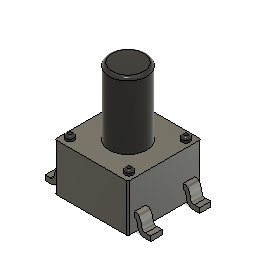
PTS 647 SK70 SMTR2 LFS v1 (Autodesk Fusion 360 design; units mm, degrees)
Autodesk Fusion 360 part; units mm, degrees
note: some values were not read from the file. Set by a fixed rule: which sketch regions a step uses.
sketch "Sketch1" plane through (0, 0, 0) normal (0, 1, 0) x (1, 0, 0)
  line L0 (-3.4, 2.1) -> (-1.85, 2.1)
  line L1 (-1.85, 2.1) -> (-1.85, 1.1)
  line L2 (-1.85, 1.1) -> (-3.4, 1.1)
  line L3 (-3.4, 1.1) -> (-3.4, 2.1)
  line L4 (0, 0) -> (0, 11.3679) construction
  line L5 (0, 11.3679) -> (0, 0) construction
  line L6 (0, 0) -> (-41.6143, 0) construction
  line L7 (3.4, 2.1) -> (1.85, 2.1)
  line L8 (1.85, 1.1) -> (3.4, 1.1)
  line L9 (1.85, 2.1) -> (1.85, 1.1)
  line L10 (3.4, 1.1) -> (3.4, 2.1)
  line L11 (-3.4, -2.1) -> (-1.85, -2.1)
  line L12 (-1.85, -2.1) -> (-1.85, -1.1)
  line L13 (3.4, -2.1) -> (1.85, -2.1)
  line L14 (-3.4, -1.1) -> (-3.4, -2.1)
  line L15 (3.4, -1.1) -> (3.4, -2.1)
  line L16 (0, 0) -> (0, -11.3679) construction
  line L17 (1.85, -1.1) -> (3.4, -1.1)
  line L18 (1.85, -2.1) -> (1.85, -1.1)
  line L19 (-1.85, -1.1) -> (-3.4, -1.1)
  line L20 (0, -11.3679) -> (0, 0) construction
  line L21 (-2.625, 2.1) -> (-2.625, 1.1) construction
  line L22 (-3.4, 1.6) -> (-1.85, 1.6) construction
  dimension "d1" = 1.85
  dimension "d2" = 3.4
  dimension "d3" = 1.1
  dimension "d4" = 2.1
  dimension "d5" = 2.625
  dimension "d6" = 1.6
  dimension "d7" = 3.7
  dimension "d8" = 6.8
  dimension "d9" = 4.2
  constraint horizontal L0
  constraint vertical L1
  constraint horizontal L2
  constraint vertical L3
  constraint coincident L4.start L5.end
  constraint vertical L4
  constraint parallel L4 L5
  constraint perpendicular L4 L6
  constraint symmetric L0.start L5 L7.start
  constraint symmetric L0.end L5 L7.end
  constraint symmetric L1.end L5 L8.start
  constraint symmetric L2.end L5 L8.end
  constraint symmetric L0.start L6 L11.start
  constraint symmetric L0.end L6 L11.end
  constraint symmetric L1.end L6 L12.end
  constraint symmetric L2.end L6 L14.start
  constraint symmetric L4.start L6 L5.end
  constraint symmetric L4.end L6 L16.end
  constraint symmetric L6 L7.start L13.start
  constraint symmetric L6 L8.end L15.start
  constraint symmetric L6 L8.start L17.start
  constraint symmetric L6 L7.end L13.end
  constraint midpoint L0 L21.start
  constraint midpoint L2 L21.end
  constraint midpoint L3 L22.start
  constraint midpoint L1 L22.end
  measures "d1" distance of L1 L5
  measures "d2" distance of L3 L4
  measures "d3" distance of L2 L6
  measures "d4" distance of L0 L6
  measures "d5" distance of L4 L21
  measures "d6" distance of L6 L22
  measures "d7" distance of L1 L9
  measures "d8" distance of L3 L10
  measures "d9" distance of L0 L11
sketch "Sketch2" plane through (0, 0, 0) normal (0, 1, 0) x (1, 0, 0)
  line L0 (-2.25, 2.25) -> (2.25, 2.25)
  line L1 (2.25, 2.25) -> (2.25, -2.25)
  line L2 (2.25, -2.25) -> (-2.25, -2.25)
  line L3 (-2.25, -2.25) -> (-2.25, 2.25)
  line L4 (0, 0) -> (4.5886, 0) construction
  line L5 (0, 0) -> (0, 2.1245) construction
  circle A0 centre (-2.15, 2.15) radius 0.1
  circle A1 centre (2.15, 2.15) radius 0.1
  circle A2 centre (2.15, -2.15) radius 0.1
  circle A3 centre (-2.15, -2.15) radius 0.1
  line L6 (-2.15, -2.15) -> (-2.15, -2.05)
  line L7 (-2.15, 2.05) -> (-2.15, 2.15)
  line L8 (-2.15, 2.15) -> (-2.05, 2.15)
  line L9 (2.05, 2.15) -> (2.15, 2.15)
  line L10 (2.15, 2.15) -> (2.15, 2.05)
  line L11 (2.15, -2.05) -> (2.15, -2.15)
  line L12 (2.15, -2.15) -> (2.05, -2.15)
  line L13 (-2.05, -2.15) -> (-2.15, -2.15)
  dimension "d10" = 2.25
  dimension "d11" = 2.25
  dimension "d12" = 2.25
  dimension "d13" = 2.25
  constraint horizontal L0
  constraint vertical L1
  constraint horizontal L2
  constraint vertical L3
  constraint coincident L4.start L5.start
  constraint horizontal L4
  constraint perpendicular L0 L5
  constraint coincident A0.centre L7.end
  constraint tangent L0 A0
  constraint coincident A1.centre L9.end
  constraint tangent L1 A1
  constraint coincident A2.centre L11.end
  constraint tangent L2 A2
  constraint coincident A3.centre L6.start
  constraint tangent L2 A3
  constraint coincident A3 L6.end
  constraint coincident A0 L7.start
  constraint collinear L6 L7
  constraint coincident A0 L8.end
  constraint coincident A1 L9.start
  constraint collinear L8 L9
  constraint coincident A1 L10.end
  constraint collinear L10 L11
  constraint coincident A2 L11.start
  constraint coincident A2 L12.end
  constraint coincident A3 L13.start
  constraint collinear L12 L13
  measures "d10" distance of L0 L4
  measures "d11" distance of L2 L4
  measures "d12" distance of L1 L5
  measures "d13" distance of L3 L5
extrude "Extrude1" add sketch "Sketch2" along normal blind 2.9 contours L0 L1 L2 L3 A0 A1 A2 A3 | A0 L7 L8 | A1 L9 L10 | A0 L7 L8 | A3 L6 L13 | A1 L9 L10 | A3 L6 L13 | A2 L11 L12 | A2 L11 L12 makes body 1
sketch "Sketch3" plane through (0, 2.9, 0) normal (0, 1, 0) x (-1, 0, 0)
  arc A0 (-2.25, -2.15) -> (-2.15, -2.25) centre (-2.15, -2.15) ccw
  line L0 (-2.15, -2.25) -> (2.15, -2.25)
  arc A1 (2.15, -2.25) -> (2.25, -2.15) centre (2.15, -2.15) ccw
  line L1 (2.25, -2.15) -> (2.25, 2.15)
  arc A2 (2.25, 2.15) -> (2.15, 2.25) centre (2.15, 2.15) ccw
  line L2 (2.15, 2.25) -> (-2.15, 2.25)
  arc A3 (-2.15, 2.25) -> (-2.25, 2.15) centre (-2.15, 2.15) ccw
  line L3 (-2.25, 2.15) -> (-2.25, -2.15)
  circle A4 centre (0, 0) radius 1.15
  dimension "d17" = 2.3
  constraint coincident A4.centre origin
  measures "d17" diameter of A4
extrude "Extrude2" add sketch "Sketch3" along normal blind 4.1 separate body contours A4 makes body 2
fillet "Fillet1" radius 0.182 1 edges at (1.0722, 7, -0.4159) on bodies 2
sketch "Sketch4" plane through (0, 0, 0) normal (0, 1, 0) x (1, 0, 0)
  arc A0 (2.25, 2.15) -> (2.15, 2.25) centre (2.15, 2.15) ccw
  line L0 (2.15, 2.25) -> (-2.15, 2.25)
  arc A1 (-2.15, 2.25) -> (-2.25, 2.15) centre (-2.15, 2.15) ccw
  line L1 (-2.25, 2.15) -> (-2.25, -2.15)
  arc A2 (-2.25, -2.15) -> (-2.15, -2.25) centre (-2.15, -2.15) ccw
  line L2 (-2.15, -2.25) -> (2.15, -2.25)
  arc A3 (2.15, -2.25) -> (2.25, -2.15) centre (2.15, -2.15) ccw
  line L3 (2.25, -2.15) -> (2.25, 2.15)
  line L4 (2.25, 1.85) -> (3.25, 1.85)
  line L5 (3.25, 1.85) -> (3.25, 1.15)
  line L6 (3.25, 1.15) -> (2.25, 1.15)
  line L7 (2.25, 1.15) -> (2.25, 1.85)
  line L8 (0, 0) -> (0, 2.7437) construction
  line L9 (0, 0) -> (3.2368, 0) construction
  line L10 (3.25, 1.5) -> (2.25, 1.5) construction
  line L11 (-2.25, 1.15) -> (-2.25, 1.85)
  line L12 (-3.25, 1.5) -> (-2.25, 1.5) construction
  line L13 (-3.25, 1.15) -> (-2.25, 1.15)
  line L14 (-2.25, 1.85) -> (-3.25, 1.85)
  line L15 (-3.25, 1.85) -> (-3.25, 1.15)
  line L16 (-3.25, -1.5) -> (-2.25, -1.5) construction
  line L17 (-3.25, -1.15) -> (-2.25, -1.15)
  line L18 (2.25, -1.85) -> (3.25, -1.85)
  line L19 (2.25, -1.15) -> (2.25, -1.85)
  line L20 (3.25, -1.5) -> (2.25, -1.5) construction
  line L21 (3.25, -1.85) -> (3.25, -1.15)
  line L22 (3.25, -1.15) -> (2.25, -1.15)
  line L23 (-2.25, -1.85) -> (-3.25, -1.85)
  line L24 (-3.25, -1.85) -> (-3.25, -1.15)
  line L25 (-2.25, -1.15) -> (-2.25, -1.85)
  dimension "d22" = 0.7
  dimension "d23" = 1.5
  dimension "d24" = 3.25
  constraint horizontal L4
  constraint vertical L5
  constraint horizontal L6
  constraint vertical L7
  constraint coincident L3 L4.start
  constraint coincident L8.start L9.start
  constraint perpendicular L0 L8
  constraint perpendicular L3 L9
  constraint midpoint L5 L10.start
  constraint midpoint L7 L10.end
  constraint perpendicular L7 L10
  constraint symmetric L4.start L8 L11.end
  constraint symmetric L4.end L8 L14.end
  constraint symmetric L5.end L8 L13.start
  constraint symmetric L6.end L8 L11.start
  constraint symmetric L8 L10.start L12.start
  constraint symmetric L8 L10.end L12.end
  constraint symmetric L4.start L9 L18.start
  constraint symmetric L4.end L9 L18.end
  constraint symmetric L5.end L9 L21.end
  constraint symmetric L6.end L9 L19.start
  constraint symmetric L9 L10.start L20.start
  constraint symmetric L9 L10.end L20.end
  constraint symmetric L9 L13.start L17.start
  constraint symmetric L9 L12.start L16.start
  constraint symmetric L9 L11.end L23.start
  constraint symmetric L9 L14.end L23.end
  constraint symmetric L9 L11.start L17.end
  constraint symmetric L9 L12.end L16.end
  measures "d22" distance of L4 L6
  measures "d23" distance of L9 L10
  measures "d24" distance of L5 L8
extrude "Extrude3" add sketch "Sketch4" along normal blind 1.1 separate body contours L3 L4 L5 L6 L7 | L3 L18 L19 L21 L22 | L1 L11 L13 L14 L15 | L1 L17 L23 L24 L25 makes body 3 at (-2.5833, 0.3667, 1.85) makes body 4 at (2.9167, 0.3667, 1.15) makes body 5 at (-2.9167, 0.3667, -1.15) makes body 6 at (2.5833, 0.3667, -1.85)
sketch "Sketch5" plane through (0, 0, 1.85) normal (0, 0, 1) x (1, 0, 0)
  line L0 (-3.25, 0) -> (-2.25, 0)
  line L1 (-2.25, 0) -> (-2.25, 1.1)
  line L2 (-2.25, 1.1) -> (-3.25, 1.1)
  line L3 (-3.25, 1.1) -> (-3.25, 0)
  spline S0 degree 5 poles (-2.25, 1.1) (-2.2628, 1.1) (-2.2878, 1.0998) (-2.3231, 1.0986) (-2.3663, 1.0951) (-2.4149, 1.0843) (-2.4595, 1.0632) (-2.5015, 1.029) (-2.5413, 0.9802) (-2.5785, 0.9184) (-2.6121, 0.8469) (-2.6407, 0.77) (-2.6638, 0.6924) (-2.6812, 0.6182) (-2.6943, 0.5503) (-2.7054, 0.4902) (-2.7173, 0.4386) (-2.7331, 0.3954) (-2.7551, 0.3605) (-2.7851, 0.3335) (-2.824, 0.3143) (-2.8625, 0.3049) (-2.8954, 0.3012) (-2.9193, 0.3001) (-2.9316, 0.3) knots 0 0 0 0 0 0 0.05 0.1 0.15 0.2 0.25 0.3 0.35 0.4 0.45 0.5 0.55 0.6 0.65 0.7 0.75 0.8 0.85 0.9 0.95 1 1 1 1 1 1
  line L4 (-2.1024, 1.1) -> (-2.3976, 1.1)
  spline S1 degree 5 poles (-2.25, 0.8) (-2.2598, 0.7991) (-2.2788, 0.7959) (-2.3051, 0.7869) (-2.3359, 0.7663) (-2.3673, 0.7261) (-2.392, 0.6717) (-2.411, 0.6043) (-2.4263, 0.5262) (-2.441, 0.4415) (-2.4588, 0.3547) (-2.4837, 0.2708) (-2.5189, 0.1943) (-2.567, 0.1286) (-2.6294, 0.0755) (-2.7063, 0.0357) (-2.7795, 0.0148) (-2.8409, 0.0051) (-2.8846, 0.0012) (-2.9072, 0) knots 0 0 0 0 0 0 0.066667 0.133333 0.2 0.266667 0.333333 0.4 0.466667 0.533333 0.6 0.666667 0.733333 0.8 0.866667 0.933333 1 1 1 1 1 1
  line L5 (-3.25, 0.3) -> (-2.9315, 0.3)
  line L6 (-2.4766, 0.3) -> (-2.25, 0.3)
  line L7 (-2.9072, 0) -> (-3.25, 0)
  line L8 (0, 0) -> (0, 0.8485)
  line L9 (2.9072, 0) -> (3.25, 0)
  line L10 (3.25, 0) -> (2.25, 0)
  spline S2 degree 5 poles (2.25, 1.1) (2.2628, 1.1) (2.2878, 1.0998) (2.3231, 1.0986) (2.3663, 1.0951) (2.4149, 1.0843) (2.4595, 1.0632) (2.5015, 1.029) (2.5413, 0.9802) (2.5785, 0.9184) (2.6121, 0.8469) (2.6407, 0.77) (2.6638, 0.6924) (2.6812, 0.6182) (2.6943, 0.5503) (2.7054, 0.4902) (2.7173, 0.4386) (2.7331, 0.3954) (2.7551, 0.3605) (2.7851, 0.3335) (2.824, 0.3143) (2.8625, 0.3049) (2.8954, 0.3012) (2.9193, 0.3001) (2.9316, 0.3) knots 0 0 0 0 0 0 0.05 0.1 0.15 0.2 0.25 0.3 0.35 0.4 0.45 0.5 0.55 0.6 0.65 0.7 0.75 0.8 0.85 0.9 0.95 1 1 1 1 1 1
  line L11 (-2.7676, 0.3019) -> (-3.0957, 0.2981)
  line L12 (2.1024, 1.1) -> (2.3976, 1.1)
  line L13 (2.7676, 0.3019) -> (3.0957, 0.2981)
  spline S3 degree 5 poles (2.25, 0.8) (2.2598, 0.7991) (2.2788, 0.7959) (2.3051, 0.7869) (2.3359, 0.7663) (2.3673, 0.7261) (2.392, 0.6717) (2.411, 0.6043) (2.4263, 0.5262) (2.441, 0.4415) (2.4588, 0.3547) (2.4837, 0.2708) (2.5189, 0.1943) (2.567, 0.1286) (2.6294, 0.0755) (2.7063, 0.0357) (2.7795, 0.0148) (2.8409, 0.0051) (2.8846, 0.0012) (2.9072, 0) knots 0 0 0 0 0 0 0.066667 0.133333 0.2 0.266667 0.333333 0.4 0.466667 0.533333 0.6 0.666667 0.733333 0.8 0.866667 0.933333 1 1 1 1 1 1
  line L14 (-2.1257, 0.8097) -> (-2.3743, 0.7903)
  line L15 (-2.7194, -0.0035) -> (-3.0951, 0.0035)
  line L16 (2.1257, 0.8097) -> (2.3743, 0.7903)
  line L17 (2.7194, -0.0035) -> (3.0951, 0.0035)
  line L18 (2.25, 0) -> (2.25, 1.1)
  line L19 (2.25, 1.1) -> (3.25, 1.1)
  line L20 (3.25, 1.1) -> (3.25, 0)
  line L21 (2.4766, 0.3) -> (2.25, 0.3)
  line L22 (3.25, 0.3) -> (2.9315, 0.3)
  point P0 (-2.4971, 1.0292)
  point P1 (-2.6664, 0.6781)
  point P2 (-2.7392, 0.3886)
  point P3 (-2.4045, 0.6237)
  point P4 (-2.515, 0.2094)
  point P5 (2.515, 0.2094)
  point P6 (2.7392, 0.3886)
  point P7 (2.4045, 0.6237)
  point P8 (2.6664, 0.6781)
  point P9 (2.4971, 1.0292)
  dimension "d27" = 0.3
  dimension "d28" = 0.3
  constraint coincident L3 L5.start
  constraint coincident L1 L6.end
  constraint perpendicular L1 L5
  constraint coincident L1.end L2.start
  constraint coincident S0.end L5
  constraint midpoint L1.end L4
  constraint coincident L2 L4.end
  constraint coincident L1 S1.start
  constraint coincident L0 S1.end
  constraint coincident S0 L5.end
  constraint coincident S1 L6.start
  constraint collinear L5 L6
  constraint coincident L0.start L3.end
  constraint coincident L8.start origin
  constraint vertical L8
  constraint midpoint S0.end L11
  constraint midpoint S1.start L14
  constraint midpoint S1.end L15
  constraint symmetric L0.start L8 L9.end
  constraint symmetric L0.end L8 L10.end
  constraint symmetric L1.end L8 S2.start
  constraint symmetric L2.end L8 L19.end
  constraint symmetric L5.start L8 L22.start
  constraint symmetric L6.end L8 L21.end
  constraint symmetric P0 L8 P9
  constraint symmetric P1 L8 P8
  constraint symmetric P2 L8 P6
  constraint symmetric S0.end L8 S2.end
  constraint symmetric L4.start L8 L12.start
  constraint symmetric L4.end L8 L12.end
  constraint symmetric S1.start L8 S3.start
  constraint symmetric P3 L8 P7
  constraint symmetric P4 L8 P5
  constraint symmetric S1.end L8 L9.start
  constraint symmetric L5.end L8 L22.end
  constraint symmetric L6.start L8 L21.start
  constraint symmetric L8 L11.start L13.start
  constraint symmetric L8 L11.end L13.end
  constraint symmetric L8 L14.start L16.start
  constraint symmetric L8 L14.end L16.end
  constraint symmetric L8 L15.start L17.start
  constraint symmetric L8 L15.end L17.end
  measures "d27" distance of L0 L5
  measures "d28" distance of L1.end S1.start
extrude "Extrude4" cut sketch "Sketch5" against normal blind 4.671 contours L0 L1 S1 L6 | L2 L3 S0 L4 L5 L11 | L1 S1 L6 | L10 S3 L18 L21 | S3 L18 L21 | S2 L12 L13 L19 L20 L22 bodies 3 4 5 6
sketch "Sketch6" plane through (0, 2.9, 0) normal (0, 1, 0) x (-1, 0, 0)
  arc A0 (-2.25, -2.15) -> (-2.15, -2.25) centre (-2.15, -2.15) ccw
  line L0 (-2.15, -2.25) -> (2.15, -2.25)
  arc A1 (2.15, -2.25) -> (2.25, -2.15) centre (2.15, -2.15) ccw
  line L1 (2.25, -2.15) -> (2.25, 2.15)
  arc A2 (2.25, 2.15) -> (2.15, 2.25) centre (2.15, 2.15) ccw
  line L2 (2.15, 2.25) -> (-2.15, 2.25)
  arc A3 (-2.15, 2.25) -> (-2.25, 2.15) centre (-2.15, 2.15) ccw
  line L3 (-2.25, 2.15) -> (-2.25, -2.15)
  line L4 (1.8149, -1.75) -> (-1.8149, -1.75)
  line L5 (-1.8149, -1.75) -> (-1.8149, 1.75)
  line L6 (-1.8149, 1.75) -> (1.8149, 1.75)
  line L7 (1.8149, 1.75) -> (1.8149, -1.75)
  line L8 (1.8149, -1.75) -> (-1.8149, 1.75) construction
  line L9 (-1.8149, -1.75) -> (1.8149, 1.75) construction
  circle A4 centre (1.8149, -1.75) radius 0.25
  circle A5 centre (-1.8149, -1.75) radius 0.25
  circle A6 centre (-1.8149, 1.75) radius 0.25
  circle A7 centre (1.8149, 1.75) radius 0.25
  dimension "d31" = 3.5
  dimension "d32" = 0.5
  dimension "d33" = 0.5
  dimension "d34" = 0.5
  dimension "d35" = 0.5
  constraint horizontal L4
  constraint perpendicular L4 L5
  constraint parallel L4 L6
  constraint parallel L5 L7
  constraint coincident L8 origin
  constraint coincident L9 origin
  constraint coincident L4.start L7.end
  constraint coincident L4.end L5.start
  constraint coincident L5.end L6.start
  constraint coincident L6.end L7.start
  measures "d31" distance of L4.end L5.end
  measures "d32" diameter of A4
  measures "d33" diameter of A5
  measures "d34" diameter of A6
  measures "d35" diameter of A7
extrude "Extrude5" add sketch "Sketch6" along normal blind 0.3 separate body contours L4 L5 A5 | L4 L5 A5 | L4 L7 A4 | L4 L7 A4 | L5 L6 A6 | L5 L6 A6 | L6 L7 A7 | L6 L7 A7 makes body 7 at (-2.0637, 3.1, -1.7251) makes body 8 at (1.5662, 3.1, -1.7251) makes body 9 at (-2.0637, 3.1, 1.7749) makes body 10 at (1.5662, 3, 1.7251)
fillet "Fillet2" radius 0.151 4 edges at (-1.5819, 3.2, -1.8404) (2.048, 3.2, -1.8404) (-1.5819, 3.2, 1.6596) (2.048, 3.2, 1.6596) on bodies 7 8 9 10
equation "d1 = ( 3.7 / 2 ) * 1 mm"
equation "d2 = ( 6.8 / 2 ) * 1 mm"
equation "d4 = ( 4.2 / 2 ) * 1 mm"
equation "d10 = ( 4.5 / 2 ) * 1 mm"
equation "d11 = d10"
equation "d12 = d10"
equation "d13 = d12"
equation "d18 = 7 mm - 2.9 mm"
equation "d23 = ( 3 / 2 ) * 1 mm"
equation "d24 = ( 6.5 / 2 ) * 1 mm"
